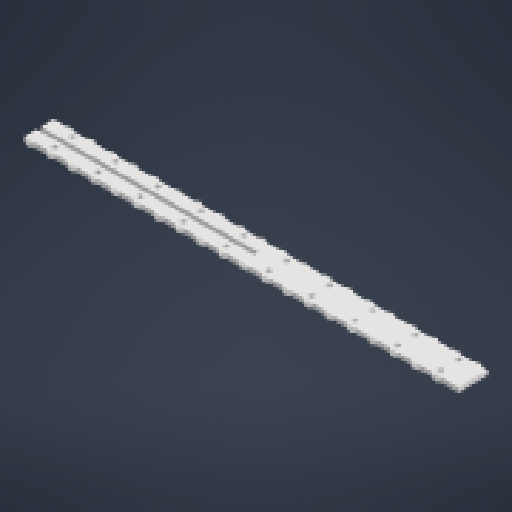
# Autodesk Inventor part: Bottom Body
Saved by Autodesk Inventor 2027 (Build 310192000, 192)
## iProperties
Created: 2026-03-26
Part Number: Bottom Body
Material: Generic
Document SubType Name: Modeling
Designer: Tueha
Density: 1 g/cm^3
Appearance: Default
Author: Tueha
Autodesk Inventor part; units mm, degrees
ref_plane "YZ Plane" through (0, 0, 0) normal (1, 0, 0) x (0, 1, 0)
ref_plane "XZ Plane" through (0, 0, 0) normal (0, 1, 0) x (-1, 0, 0)
ref_plane "XY Plane" through (0, 0, 0) normal (0, 0, 1) x (1, 0, 0)
sketch "Sketch1" plane through (0, 0, 0) normal (0, 1, 0) x (-1, 0, 0)
  line L0 (0, 0) -> (57.6, 0)
  line L1 (57.6, 0) -> (57.6, -39.8)
  line L2 (57.6, -39.8) -> (0, -39.8)
  line L3 (0, -39.8) -> (0, 0)
  circle A0 centre (7.2, -39.8) radius 1
  circle A1 centre (36, -39.8) radius 1
  circle A2 centre (21.6, 0) radius 1
  circle A3 centre (50.4, 0) radius 1
  line L4 (22.2, -10.9) -> (28.2, -10.9)
  line L5 (28.2, -10.9) -> (28.2, -4.9)
  line L6 (28.2, -4.9) -> (22.2, -4.9)
  line L7 (22.2, -4.9) -> (22.2, -10.9)
  line L8 (22.2, -34.9) -> (28.2, -34.9)
  line L9 (28.2, -34.9) -> (28.2, -28.9)
  line L10 (28.2, -28.9) -> (22.2, -28.9)
  line L11 (22.2, -28.9) -> (22.2, -34.9)
  line L12 (20.6, 0) -> (20.6, 3)
  line L13 (22.6, 0) -> (22.6, 3)
  line L14 (22.6, 3) -> (27.7962, 0)
  line L15 (20.6, 3) -> (15.4038, 0)
  line L16 (49.4, 3) -> (44.2038, 0)
  line L17 (49.4, 0) -> (49.4, 3)
  line L18 (51.4, 0) -> (51.4, 3)
  line L19 (51.4, 3) -> (56.5962, 0)
  line L20 (37, -39.8) -> (37, -42.8)
  line L21 (37, -42.8) -> (42.1962, -39.8)
  line L22 (35, -39.8) -> (35, -42.8)
  line L23 (35, -42.8) -> (29.8038, -39.8)
  line L24 (8.2, -39.8) -> (8.2, -42.8)
  line L25 (8.2, -42.8) -> (13.3962, -39.8)
  line L26 (6.2, -39.8) -> (6.2, -42.8)
  line L27 (6.2, -42.8) -> (1.0038, -39.8)
  point P0 (28.2, -7.9)
  point P1 (28.2, -31.9)
  point P2 (25.2, -34.9)
  point P3 (8.2, -39.8)
  point P4 (6.2, -39.8)
  point P5 (56.5962, 0)
  point P6 (51.4, 0)
  point P7 (49.4, 0)
  point P8 (44.2038, 0)
  dimension "hd" = 57.6
  dimension "Length" = 39.8
  dimension "d2" = 2
  dimension "d4" = 2
  dimension "d5" = 28.8
  dimension "d7" = 2
  dimension "d8" = 21.6
  dimension "d10" = 0
  dimension "d11" = 0
  dimension "d12" = 2
  dimension "d13" = 0
  dimension "d14" = 28.8
  dimension "d15" = 39.8
  dimension "d16" = 7.2
  dimension "d43" = 6
  dimension "d44" = 6
  dimension "d47" = 4.9
  dimension "d48" = 29.4
  dimension "d49" = 6
  dimension "d50" = 6
  dimension "d51" = 4.9
  dimension "d56" = 29.4
  dimension "d57" = 3
  dimension "d58" = 6
  dimension "d59" = 3
  dimension "d60" = 6
  dimension "d63" = 28.8
  dimension "d68" = 3
  dimension "d69" = 6
  dimension "d72" = 28.8
  constraints: 56 end point, 7 point on line, 6 parallel, 5 horizontal, 4 centre point, 4 point on circle, 3 midpoint, 3 perpendicular, 3 tangent, 1 vertical, 20 other
  measures "hd" distance of L1.end L2.end
  measures "Length" distance of L0.end L1.end
  measures "d2" diameter of A0
  measures "d4" diameter of A1
  measures "d5" distance of A0.centre A1.centre
  measures "d7" diameter of A2
  measures "d8" distance from line of L3 A2.centre
  measures "d10" distance from line of L2 A0.centre
  measures "d11" vertical distance of A0.centre A1.centre
  measures "d12" diameter of A3
  measures "d13" vertical distance of A3.centre A2.centre
  measures "d14" distance of A2.centre A3.centre
  measures "d15" vertical distance of A2.centre A0.centre
  measures "d16" distance from line of L3 A0.centre
  measures "d43" distance of L4.end L5.end
  measures "d44" distance of L4.start L4.end
  measures "d47" distance between parallel lines of L0 L6
  measures "d48" distance from line of L1 point (28.2, -7.9)
  measures "d49" distance of L8.end L10.start
  measures "d50" distance of L11.end L8.end
  measures "d51" distance from line of L2 point (25.2, -34.9)
  measures "d56" distance between parallel lines of L1 L9
  measures "d57" distance of L12.start L12.end
  measures "d58" distance of L13.end L14.end
  measures "d59" distance of L13.start L13.end
  measures "d60" distance of L12.end L15.end
  measures "d63" distance of L12.end L16.start
  measures "d68" distance of L20.start L20.end
  measures "d69" distance of L20.end L21.end
  measures "d72" distance of L20.start L24.start
extrude "Extrusion1" add sketch "Sketch1" along normal blind 6 contours L0 A2 A3 L1 L2 A1 A0 L3 | L15 L12 L0 | L2 L26 L27 | L13 L14 L0 | L2 L25 L24 | L16 L17 L0 | L2 L22 L23 | L18 L19 L0 | L2 L21 L20 | L7 L6 L5 L4 | L11 L10 L9 L8
pattern_linear "Rectangular Pattern2" count 10 spacing 57.6 along (1, 0, 0) of "Extrusion1"
sketch "Sketch7" plane through (0, 6, 0) normal (0, 1, 0) x (1, 0, 0)
  line L0 (-57.6, 22.9) -> (234, 22.9)
  line L1 (234, 22.9) -> (234, 16.9)
  line L2 (234, 16.9) -> (-57.6, 16.9)
  line L3 (-57.6, 16.9) -> (-57.6, 22.9)
  line L4 (-57.6, 39.8) -> (-57.6, 0) projected
  line L5 (-42.1962, 39.8) -> (-57.6, 39.8) projected
  point P0 (0, 0)
  point P1 (-37.7321, 39.8)
  dimension "d35" = 6
  dimension "d36" = 0
  dimension "d37" = 16.9
  dimension "d38" = 291.6
  constraints: 8 end point, 2 parallel, 1 horizontal, 1 perpendicular
  measures "d35" distance of L2.end L0.start
  measures "d36" distance between parallel lines of L4 L3
  measures "d37" distance between parallel lines of L5 L0
  measures "d38" distance of L1.end L2.end
extrude "Extrusion4" cut sketch "Sketch7" against normal blind 9.175
sketch "Sketch8" plane through (518.4, 0, 0) normal (1, 0, 0) x (0, 0, -1)
  line L0 (38.8, 6) -> (39.8, 6) projected
  line L1 (0, 0) -> (39.8, 0)
  line L2 (39.8, 0) -> (39.8, 6)
  line L3 (39.8, 6) -> (0, 6)
  line L4 (0, 6) -> (0, 0)
  point P0 (39.3, 6)
  constraints: 8 end point, 2 parallel, 1 horizontal, 1 perpendicular
extrude "Extrusion5" add sketch "Sketch8" along normal blind 7.2
extrude "Extrusion6" cut sketch "Sketch1" along normal blind 9.175 contours L7 L6 L5 L4 | L11 L10 L9 L8
pattern_linear "Rectangular Pattern3" count 10 spacing 57.6 along (1, 0, 0) of "Extrusion6"
sketch "Sketch10" plane through (-57.6, 0, 0) normal (0, 0, 1) x (1, 0, 0)
  line L0 (0, 6) -> (291.6, 6) projected
  line L1 (0, 0) -> (291.6, 0) projected
  line L2 (6.2708, 6) -> (0, 6)
  line L3 (0, 6) -> (0, 0)
  line L4 (0, 0) -> (6.2708, 0)
  line L5 (6.2708, 0) -> (6.2708, 6)
  point P0 (57.6, 0)
  constraints: 8 end point, 2 parallel, 1 horizontal, 1 perpendicular, 1 point on line
extrude "Extrusion7" cut sketch "Sketch10" along normal blind 6
equation "\"d5\" = 0.5 * hd"
equation "\"d8\" = 0.5 * d5 + d16"
equation "\"d10\" = -0.5 * d + 0.5 * Length"
equation "\"d14\" = d5"
equation "\"d15\" = d"
equation "\"d16\" = 0.125 * hd"
equation "\"d51\" = d47"
equation "\"d56\" = d48"
equation "\"d34\" = hd"
equation "\"d38\" = 5.0625 * hd"
equation "\"d41\" = 0.125 * hd"
equation "\"d55\" = hd"
equation "\"d\" = 39.8"
body "Solid1"
